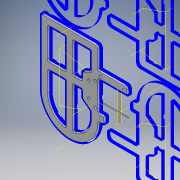
# Autodesk Inventor part: base_head
Saved by Autodesk Inventor 2018 (Build 220112000, 112)
## iProperties
Created: 2018-04-23
Part Number: base_head
Material: Aluminum 6061
Document SubType Name: Modeling
Designer: medrimonia
Density: 2.7 g/cm^3
Appearance: Aluminum - Flat
Mass: 20.1361 g
Surface Area: 72.9531 cm^2
Volume: 7.45782 cm^3
Vendor: Rhoban
Author: medrimonia
Autodesk Inventor part; units mm, degrees
ref_plane "YZ Plane" through (0, 0, 0) normal (1, 0, 0) x (0, 1, 0)
ref_plane "XZ Plane" through (0, 0, 0) normal (0, 1, 0) x (-1, 0, 0)
ref_plane "XY Plane" through (0, 0, 0) normal (0, 0, 1) x (1, 0, 0)
sketch "Sketch1" plane through (0, 0, 0) normal (0, 1, 0) x (-1, 0, 0)
  line L0 (0, 0) -> (0, -14.8)
  line L1 (0, -14.8) -> (-5.8, -14.8)
  line L2 (-5.8, -14.8) -> (-5.8, -20.8)
  line L3 (-5.8, -20.8) -> (0, -20.8)
  line L4 (0, 0) -> (0, 14.8)
  line L5 (0, 14.8) -> (-27.8, 14.8)
  line L6 (-27.8, 14.8) -> (-27.8, 20.8)
  line L7 (-27.8, 20.8) -> (0, 20.8)
  line L8 (0, 20.8) -> (0, 40.8)
  line L9 (0, 40.8) -> (54, 40.8)
  line L10 (0, -20.8) -> (0, -21.8)
  line L11 (54, 40.8) -> (54, -21.8)
  arc A0 (0, -21.8) -> (54, -21.8) centre (27, -21.8) ccw
  line L12 (-27.8, 17.3) -> (2.5, 17.3) construction
  line L13 (2.5, 17.3) -> (2.5, -17.3) construction
  line L14 (2.5, -17.3) -> (-5.8, -17.3) construction
  line L15 (0, 0) -> (2.5, 0) construction
  line L16 (2.5, 0) -> (8.5, 0) construction
  line L17 (8.5, -6.35) -> (8.5, 8.35) construction
  line L18 (-27.8, 14.8) -> (-5.8, -14.8) construction
  line L19 (-16.8, 0) -> (-21.8, 0) construction
  point P0 (-2.8, -17.3)
  point P1 (-2.8, 17.3)
  point P2 (-24.8, 17.3)
  point P3 (2.5, 11)
  point P4 (2.5, -11)
  dimension "d0" = 20
  dimension "d1" = 6
  dimension "d2" = 6
  dimension "d4" = 54
  dimension "d5" = 1
  dimension "d7" = 2.5
  dimension "d8" = 2.5
  dimension "d9" = 5.3
  dimension "d10" = 3
  dimension "d11" = 34.6
  dimension "d12" = 11
  dimension "d13" = 11
  dimension "d14" = 5.3
  dimension "d15" = 22
  dimension "d16" = 3
  dimension "d19" = 6
  dimension "d20" = 14.7
  dimension "d21" = 6.35
  dimension "d53" = 5
  constraints: 40 end point, 11 point on line, 9 perpendicular, 5 vertical, 4 horizontal, 3 coincident, 3 midpoint, 2 point on circle, 2 tangent, 1 centre point, 1 collinear
  measures "d0" distance of L7.end L8.end
  measures "d1" distance of L1.end L2.end
  measures "d2" distance of L5.end L6.end
  measures "d4" distance of L8.end L9.end
  measures "d5" distance from line of A0.centre L3
  measures "d7" distance of L0.start L15.end
  measures "d8" distance between parallel lines of L1 L14
  measures "d9" distance from line of L13 point (-2.8, -17.3)
  measures "d10" distance from line of point (-2.8, -17.3) L2
  measures "d11" distance between parallel lines of L12 L14
  measures "d12" distance from line of L15 point (2.5, -11)
  measures "d13" distance from line of L15 point (2.5, 11)
  measures "d14" distance from line of L13 point (-2.8, 17.3)
  measures "d15" distance of point (-24.8, 17.3) point (-2.8, 17.3)
  measures "d16" distance from line of point (-24.8, 17.3) L6
  measures "d19" distance of L15.end L16.end
  measures "d20" distance of L17.start L17.end
  measures "d21" distance from line of L16 L17.start
  measures "d53" distance of L19.start L19.end
extrude "Extrusion1" add sketch "Sketch1" along normal blind 3
hole "Hole1" at (2.8, 0, -17.3) at (2.8, 0, 17.3) at (24.8, 0, 17.3) at (-2.5, 0, 11) at (-2.5, 0, -11) at (-8.5, 0, 8.35) at (-8.5, 0, -6.35) direction (0, 1, 0) diameter 2.5 end through all
fillet "ManufacturingFillet" radius 1.5 4 edges at (0, 1.5, -20.8) (0, 1.5, -14.8) (0, 1.5, 14.8) (0, 1.5, 20.8)
fillet "Fillet2" radius 2 4 edges at (5.8, 1.5, -20.8) (27.8, 1.5, 20.8) (0, 1.5, 40.8) (-54, 1.5, 40.8)
sketch "InteriorSketch" plane through (0, 3, 0) normal (0, 1, 0) x (1, 0, 0)
  arc A0 (-54, -38.8) -> (-52, -40.8) centre (-52, -38.8) ccw projected
  line L0 (-52, -40.8) -> (-2, -40.8) projected
  arc A1 (-2, -40.8) -> (0, -38.8) centre (-2, -38.8) ccw projected
  line L1 (0, -38.8) -> (0, -22.3) projected
  arc A2 (1.5, -20.8) -> (0, -22.3) centre (1.5, -22.3) ccw projected
  line L2 (1.5, -20.8) -> (25.8, -20.8) projected
  arc A3 (25.8, -20.8) -> (27.8, -18.8) centre (25.8, -18.8) ccw projected
  line L3 (27.8, -18.8) -> (27.8, -14.8) projected
  line L4 (27.8, -14.8) -> (1.5, -14.8) projected
  arc A4 (0, -13.3) -> (1.5, -14.8) centre (1.5, -13.3) ccw projected
  line L5 (0, -13.3) -> (0, 13.3) projected
  arc A5 (1.5, 14.8) -> (0, 13.3) centre (1.5, 13.3) ccw projected
  line L6 (1.5, 14.8) -> (5.8, 14.8) projected
  line L7 (5.8, 14.8) -> (5.8, 18.8) projected
  arc A6 (5.8, 18.8) -> (3.8, 20.8) centre (3.8, 18.8) ccw projected
  line L8 (3.8, 20.8) -> (1.4956, 20.8) projected
  arc A7 (-0.0042, 22.2737) -> (1.4956, 20.8) centre (1.4956, 22.3) ccw projected
  arc A8 (-0.0042, 22.2737) -> (-54, 21.8) centre (-27, 21.8) ccw projected
  line L9 (-54, 21.8) -> (-54, -38.8) projected
  circle A9 centre (-8.5, -8.35) radius 1.25 projected
  circle A10 centre (-2.5, -11) radius 1.25 projected
  circle A11 centre (2.8, -17.3) radius 1.25 projected
  circle A12 centre (2.8, 17.3) radius 1.25 projected
  circle A13 centre (24.8, -17.3) radius 1.25 projected
  circle A14 centre (-2.5, 11) radius 1.25 projected
  circle A15 centre (-8.5, 6.35) radius 1.25 projected
  line L10 (-14.5, 9.2909) -> (-14.5, -12.2592)
  line L11 (-14.5, -12.2592) -> (-6, -16.0133)
  line L12 (-6, -16.0133) -> (-6, -34.8)
  line L13 (-6, -34.8) -> (-48, -34.8)
  circle A16 centre (-2.5, 11) radius 1.25 construction
  line L14 (-8.5, 6.35) -> (-2.5, 11) construction
  line L15 (-8.5, -8.35) -> (-2.5, -11) construction
  line L16 (-14.5, 9.2909) -> (-6, 15.8784)
  line L17 (-6, 15.8784) -> (-6, 21.8)
  line L18 (-6, 15.8784) -> (-6, 21.8)
  arc A17 (-6, 21.8) -> (-48, 21.8) centre (-27, 21.8) ccw
  line L19 (-48, 21.8) -> (-48, -34.8)
  line L20 (-6, 21.8) -> (-48, 21.8) construction
  line L21 (-27, -34.8) -> (-27, 42.8) construction
  line L22 (-14.5, -1.4841) -> (-48, -1.4841) construction
  line L23 (-14.5, 1.5159) -> (-24, 1.5159)
  line L24 (-24, 1.5159) -> (-24, 42.5846)
  line L25 (-30, 42.5846) -> (-30, 1.5159)
  line L26 (-30, 1.5159) -> (-48, 1.5159)
  line L27 (-48, -4.4841) -> (-30, -4.4841)
  line L28 (-30, -4.4841) -> (-30, -34.8)
  line L29 (-14.5, -4.4841) -> (-24, -4.4841)
  line L30 (-24, -4.4841) -> (-24, -34.8)
  line L31 (-30, 1.5159) -> (-24, 1.5159) construction
  line L32 (-30, 1.5159) -> (-30, -4.4841) construction
  point P0 (0, 0)
  point P1 (-14.5, -1.4841)
  point P2 (-27, -1.4841)
  point P3 (-30, -1.4841)
  point P4 (-27, 1.5159)
  dimension "d31" = 6
  dimension "d32" = 6
  dimension "d34" = 6
  dimension "d38" = 6
  dimension "d39" = 6
  dimension "d44" = 6
  dimension "d48" = 6
  dimension "d49" = 6
  constraints: 46 end point, 15 point on line, 7 perpendicular, 6 midpoint, 6 parallel, 5 point on circle, 3 vertical, 2 coincident, 2 collinear, 2 horizontal, 1 centre point, 1 tangent
  measures "d31" distance between parallel lines of L11 L15
  measures "d32" distance from line of L10 L15.start
  measures "d34" distance between parallel lines of L14 L16
  measures "d38" distance between parallel lines of L1 L12
  measures "d39" distance between parallel lines of L0 L13
  measures "d44" distance between parallel lines of L5 L17
  measures "d48" distance between parallel lines of L29 L23
  measures "d49" distance between parallel lines of L30 L28
extrude "Extrusion3" cut sketch "InteriorSketch" against normal through all contours L10 L23 L24 A17 L17 L16 | L10 L11 L12 L13 L30 L29 | L25 L26 L19 A17 | L13 L19 L27 L28
fillet "Fillet3" radius 1.5 18 edges at (-24, 1.5, 34.8) (-6, 1.5, 34.8) (-24, 1.5, 4.4841) (-14.5, 1.5, 4.4841) (-6, 1.5, 16.0133) (-14.5, 1.5, 12.2592) (-14.5, 1.5, -9.2909) (-6, 1.5, -15.8784) (-24, 1.5, -42.5846) (-14.5, 1.5, -1.5159) (-24, 1.5, -1.5159) (-30, 1.5, -1.5159) (-30, 1.5, 4.4841) (-30, 1.5, 34.8) (-48, 1.5, 34.8) (-48, 1.5, 4.4841) (-48, 1.5, -1.5159) (-30, 1.5, -42.5846)
ref_plane "Work Plane3" through (19, 0, 13.3) normal (1, 0, 0) x (0, 0, -1)
ref_plane "Work Plane4" through (27.8, 0, -5.2) normal (0, 0, -1) x (-1, 0, 0)
equation "\"d0\" = head_back_length"
equation "\"d1\" = fix_width"
equation "\"d2\" = fix_width"
equation "\"d4\" = head_height"
equation "\"d5\" = head_forward - 0.5 * head_height"
equation "\"d7\" = hole_2_intern"
equation "\"d8\" = hole_2_intern"
equation "\"d9\" = hole_side_2_hole_top"
equation "\"d10\" = hole_2_extern"
equation "\"d11\" = side_2_side_hole"
equation "\"d12\" = 0.5 * hole_2_hole"
equation "\"d13\" = 0.5 * hole_2_hole"
equation "\"d14\" = hole_side_2_hole_top"
equation "\"d15\" = hole_2_hole"
equation "\"d16\" = hole_2_extern"
equation "\"d19\" = camera_holes_offset_z"
equation "\"d20\" = camera_holes_dist"
equation "\"d21\" = 0.5 * camera_holes_dist - camera_holes_offset_x"
equation "\"d17\" = plate_thickness"
equation "\"d31\" = structure_width"
equation "\"d32\" = structure_width"
equation "\"d34\" = structure_width"
equation "\"d38\" = structure_width"
equation "\"d39\" = structure_width"
equation "\"d44\" = structure_width"
equation "\"d48\" = structure_width"
equation "\"d49\" = structure_width"
equation "\"head_back_length\" = 20"
equation "\"head_height\" = 54"
equation "\"head_forward\" = 28"
equation "\"fix_width\" = 6"
equation "\"fix_2_fix\" = 29.1"
equation "\"hole_2_intern\" = hole_2_servo - fix_2_servo_margin"
equation "\"fix_2_servo_margin\" = 0.3"
equation "\"hole_2_servo\" = 2.8"
equation "\"side_2_side_hole\" = 34.6"
equation "\"hole_side_2_hole_top\" = 5.3"
equation "\"hole_2_extern\" = 3"
equation "\"hole_2_hole\" = 22"
equation "\"plate_thickness\" = 3"
equation "\"camera_holes_offset_z\" = 6"
equation "\"camera_holes_dist\" = 14.7"
equation "\"camera_holes_offset_x\" = 1"
equation "\"structure_width\" = 6"
body "Solid1"
